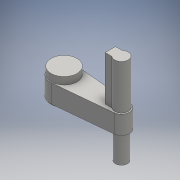
# Autodesk Inventor part: 2
Saved by Autodesk Inventor 2016 (Build 200138000, 138)
## iProperties
Created: 2015-12-17
Part Number: 2
Material: Generic
Document SubType Name: Modeling
Designer: ajshort
Density: 1 g/cm^3
Appearance: Default
Author: ajshort
Autodesk Inventor part; units mm, degrees
ref_plane "YZ Plane" through (0, 0, 0) normal (1, 0, 0) x (0, 1, 0)
ref_plane "XZ Plane" through (0, 0, 0) normal (0, 1, 0) x (-1, 0, 0)
ref_plane "XY Plane" through (0, 0, 0) normal (0, 0, 1) x (1, 0, 0)
sketch "Sketch1" plane through (0, 0, 0) normal (0, 0, 1) x (1, 0, 0)
  circle A0 centre (0, 0) radius 85
  dimension "d0" = 170
  constraints: 1 centre point, 1 coincident
  measures "d0" diameter of A0
extrude "Extrusion1" add sketch "Sketch1" along normal blind 6
sketch "Sketch2" plane through (0, 0, 6) normal (0, 0, 1) x (1, 0, 0)
  circle A0 centre (0, 0) radius 89 construction
  circle A1 centre (375, 0) radius 53 construction
  line L0 (8.544, 88.5889) -> (380.088, 52.7552)
  line L1 (8.544, -88.5889) -> (380.088, -52.7552)
  arc A2 (8.544, 88.5889) -> (8.544, -88.5889) centre (0, 0) ccw
  arc A3 (380.088, -52.7552) -> (380.088, 52.7552) centre (375, 0) ccw
  dimension "d3" = 178
  dimension "d4" = 106
  dimension "d5" = 375
  constraints: 8 point on circle, 4 centre point, 4 end point, 4 tangent, 3 coincident, 1 horizontal alignment
  measures "d3" diameter of A0
  measures "d4" diameter of A1
  measures "d5" distance of A1.centre point (0, 0)
extrude "Extrusion2" add sketch "Sketch2" along normal blind 121
sketch "Sketch3" plane through (0, 0, 127) normal (0, 0, 1) x (1, 0, 0)
  circle A0 centre (0, 0) radius 85
  dimension "d8" = 170
  constraints: 1 centre point, 1 coincident
  measures "d8" diameter of A0
extrude "Extrusion3" add sketch "Sketch3" along normal blind 48
sketch "Sketch4" plane through (0, 0, 127) normal (0, 0, 1) x (1, 0, 0)
  arc A0 (380.088, -52.7552) -> (380.088, 52.7552) centre (375, 0) ccw construction
  circle A1 centre (375, 0) radius 44.5 construction
  line L0 (302.5, 33.375) -> (302.5, -33.375)
  line L1 (302.5, 33.375) -> (345.566, 33.375)
  line L2 (302.5, -33.375) -> (345.566, -33.375)
  arc A2 (345.566, -33.375) -> (345.566, 33.375) centre (375, 0) ccw
  point P0 (0, 0)
  point P1 (302.5, 0)
  dimension "d11" = 89
  dimension "d12" = 66.75
  dimension "d13" = 72.5
  constraints: 6 end point, 4 point on circle, 2 centre point, 2 coincident, 2 horizontal, 1 horizontal alignment, 1 midpoint, 1 vertical
  measures "d11" diameter of A1
  measures "d12" distance of L0.start L0.end
  measures "d13" distance from line of A0.centre L0
extrude "Extrusion4" add sketch "Sketch4" along normal blind 292
sketch "Sketch5" plane through (0, 0, 6) normal (0, 0, -1) x (-1, 0, 0)
  arc A0 (-380.088, 52.7552) -> (-380.088, -52.7552) centre (-375, 0) ccw construction
  circle A1 centre (-375, 0) radius 39.5
  point P0 (0, 0)
  dimension "d16" = 79
  constraints: 1 centre point, 1 coincident
  measures "d16" diameter of A1
extrude "Extrusion5" add sketch "Sketch5" along normal blind 177.92
body "Solid1"
